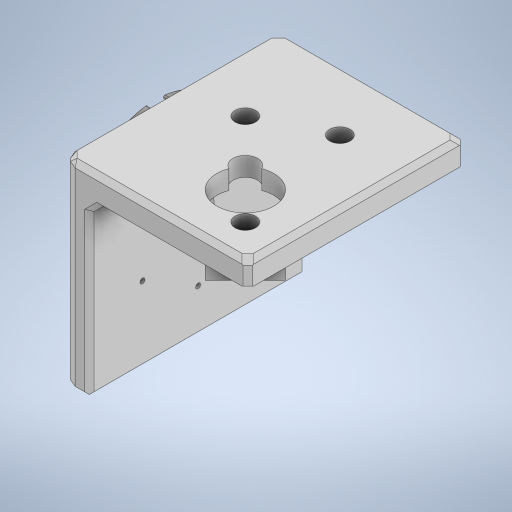
# Autodesk Inventor part: End_Effecto_Base
Saved by Autodesk Inventor 2023 (Build 270158000, 158)
## iProperties
Created: 2025-02-17
Part Number: End_Effecto_Base
Material: Generic
Document SubType Name: Modeling
Designer: Swoby
Density: 1 g/cm^3
Appearance: Default
Author: Swoby
Autodesk Inventor part; units mm, degrees
ref_plane "YZ Plane" through (0, 0, 0) normal (1, 0, 0) x (0, 1, 0)
ref_plane "XZ Plane" through (0, 0, 0) normal (0, 1, 0) x (-1, 0, 0)
ref_plane "XY Plane" through (0, 0, 0) normal (0, 0, 1) x (1, 0, 0)
sketch "Sketch1" plane through (0, 0, 0) normal (0, 0, 1) x (1, 0, 0)
  line L0 (0, 0) -> (-46, 0)
  line L1 (-46, 0) -> (-46, -38)
  line L2 (-46, -38) -> (-40, -38)
  line L3 (-40, -38) -> (-40, -6)
  line L4 (-40, -6) -> (0, -6)
  line L5 (0, -6) -> (0, 0)
  line L6 (-46, -38) -> (0, -38)
  line L7 (0, -38) -> (0, -42)
  line L8 (0, -42) -> (-46, -42)
  line L9 (-46, -42) -> (-46, -38)
  dimension "d0" = 38
  dimension "d1" = 40
  dimension "d2" = 6
  dimension "d3" = 6
  dimension "d62" = 4
  dimension "d63" = 32
  constraints: 20 end point, 6 perpendicular, 2 horizontal, 2 parallel, 1 collinear
  measures "d0" distance of L0.end L1.end
  measures "d1" distance of L3.end L4.end
  measures "d2" distance between parallel lines of L4 L0
  measures "d3" distance between parallel lines of L1 L3
  measures "d62" distance of L6.end L7.end
  measures "d63" distance between parallel lines of L4 L6
extrude "Extrusion1" add sketch "Sketch1" along normal blind 46
sketch "Sketch2" plane through (-46, 0, 0) normal (0, 1, 0) x (1, 0, 0)
  line L0 (46, 0) -> (0, 0) projected
  line L1 (0, 0) -> (0, -46) projected
  line L2 (46, -46) -> (0, -46) projected
  line L3 (46, 0) -> (46, -46) projected
  line L4 (26, 0) -> (26, -46) construction
  line L5 (46, -23) -> (26, -23) construction
  point P0 (26, -13)
  point P1 (26, -33)
  dimension "d6" = 20
  dimension "d7" = 10
  dimension "d8" = 10
  constraints: 4 end point, 4 point on line, 2 midpoint, 1 perpendicular
  measures "d6" distance between parallel lines of L4 L3
  measures "d7" distance from line of L5 point (26, -13)
  measures "d8" distance from line of point (26, -33) L5
sketch "Sketch3" plane through (-40, -6, 0) normal (0, -1, 0) x (1, 0, 0)
  circle A0 centre (20, 33) radius 6
  circle A1 centre (15.5452, 28.5452) radius 2.6
  line L0 (24.2426, 37.2426) -> (13.7067, 26.7067) construction
  line L1 (28.4853, 33) -> (20, 41.4853)
  line L2 (20, 41.4853) -> (3.9487, 25.434)
  line L3 (3.9487, 25.434) -> (12.434, 16.9487)
  line L4 (12.434, 16.9487) -> (28.4853, 33)
  line L5 (20, 33) -> (26, 33) construction
  line L6 (0, 0) -> (40, 0) projected
  line L7 (40, 0) -> (40, 46) projected
  line L8 (0, 46) -> (40, 46) projected
  line L9 (0, 0) -> (0, 46) projected
  point P0 (17.8741, 27.3892)
  point P1 (14.3892, 30.8741)
  point P2 (20, 13)
  dimension "d10" = 5.2
  dimension "d9" = 12
  dimension "d11" = 14.9
  dimension "d12" = 22.7
  dimension "d13" = 12
  dimension "d26" = 135
  constraints: 12 end point, 3 parallel, 2 point on circle, 2 point on line, 2 tangent, 1 centre point, 1 coincident, 1 horizontal, 1 perpendicular, 3 other
  measures "d9" diameter of A0
  measures "d11" distance of L0.start L0.end
  measures "d12" distance of L1.end L2.end
  measures "d13" distance of L2.end L3.end
  measures "d26" angle of L0 L5
extrude "Extrusion2" cut sketch "Sketch3" against normal through all contours A0 A1 | A1 A0 | A0 A1
extrude "Extrusion3" cut sketch "Sketch3" against normal blind 2 contours A0 A1 | A0 L1 L4 | A0 L2 L1 | L4 L3 L2 A0 A1 | A1 A0 | A0 A1
sketch "Sketch4" plane through (-40, -6, 0) normal (0, -1, 0) x (1, 0, 0)
  line L0 (3.9487, 25.434) -> (20, 41.4853) projected
  line L1 (20, 41.4853) -> (28.4853, 33) projected
  line L2 (28.4853, 33) -> (12.434, 16.9487) projected
  line L3 (12.434, 16.9487) -> (3.9487, 25.434) projected
  line L4 (0, 0) -> (40, 0) projected
  line L5 (40, 0) -> (40, 46) projected
  line L6 (0, 46) -> (40, 46) projected
  line L7 (0, 0) -> (0, 46) projected
  line L8 (28.4853, 33) -> (20, 41.4853)
  line L9 (3.9487, 25.434) -> (12.434, 16.9487)
  line L10 (12.434, 16.9487) -> (9.1106, 13.6253)
  line L11 (9.1106, 13.6253) -> (0.6253, 22.1106)
  line L12 (0.6253, 22.1106) -> (3.9487, 25.434)
  line L13 (28.4853, 33) -> (31.8087, 36.3234)
  line L14 (31.8087, 36.3234) -> (23.3234, 44.8087)
  line L15 (23.3234, 44.8087) -> (20, 41.4853)
  line L16 (31.8087, 36.3234) -> (20, 41.4853) construction
  line L17 (23.3234, 44.8087) -> (28.4853, 33) construction
  line L18 (12.434, 16.9487) -> (0.6253, 22.1106) construction
  line L19 (3.9487, 25.434) -> (9.1106, 13.6253) construction
  circle A0 centre (25.9043, 38.9043) radius 2.15
  circle A1 centre (6.5296, 19.5296) radius 2.15
  circle A2 centre (20, 13) radius 2.15
  circle A3 centre (20, 13) radius 4
  line L20 (23.3234, 44.8087) -> (24.0305, 45.5158)
  line L21 (24.0305, 45.5158) -> (32.5158, 37.0305)
  line L22 (32.5158, 37.0305) -> (31.8087, 36.3234)
  line L23 (0.6253, 22.1106) -> (0, 21.4853)
  line L24 (0, 21.4853) -> (0, 21.3216)
  line L25 (0, 21.3216) -> (8.4034, 12.9182)
  line L26 (8.4034, 12.9182) -> (9.1106, 13.6253)
  dimension "d28" = 4.7
  dimension "d29" = 4.7
  dimension "d30" = 12
  dimension "d31" = 4.3
  dimension "d32" = 4.3
  dimension "d35" = 4.3
  dimension "d36" = 8
  dimension "d76" = 1
  dimension "d77" = 1
  constraints: 38 end point, 6 collinear, 6 perpendicular, 4 centre point, 3 point on line, 2 coincident, 2 midpoint, 1 parallel
  measures "d28" distance of L2.end L10.end
  measures "d29" distance of L1.end L13.end
  measures "d30" distance of L13.end L14.end
  measures "d31" diameter of A0
  measures "d32" diameter of A1
  measures "d35" diameter of A2
  measures "d36" diameter of A3
  measures "d76" distance between parallel lines of L21 L14
  measures "d77" distance of L25.end L10.end
extrude "Extrusion4" add sketch "Sketch4" along normal blind 2.3 contours L3 L10 L11 L12 | L15 L14 L13 L1 | L11 L26 L25 L7 L23 | L20 L21 L22 L14 | A3
sketch "Sketch5" plane through (-20, -6, 41.35) normal (0, -1, 0) x (1, 0, 0)
  circle A0 centre (5.9043, -2.4457) radius 2.15 projected
  circle A1 centre (-13.4704, -21.8204) radius 2.15 projected
  circle A2 centre (0, -28.35) radius 2.15 projected
extrude "Extrusion5" cut sketch "Sketch5" against normal through all
sketch "Sketch6" plane through (-46, -38, 0) normal (-1, 0, 0) x (0, 0, 1)
  line L0 (0, 38) -> (0, 0) projected
  line L1 (0, 0) -> (46, 0) projected
  line L2 (46, 38) -> (46, 0) projected
  line L3 (0, 38) -> (46, 38) projected
  line L4 (0, 38) -> (46, 0) construction
  line L5 (0, 0) -> (46, 38) construction
  arc A0 (20.5564, 4.8718) -> (23, 2.9) centre (23, 5.4) ccw
  arc A1 (9.057, 10.95) -> (11.9864, 9.8197) centre (11.2221, 12.2) ccw
  line L6 (23, 2.9) -> (23, 19) construction
  line L7 (23, 19) -> (9.057, 10.95) construction
  circle A2 centre (23, 19) radius 8 construction
  line L8 (23, 19) -> (19, 12.0718) construction
  line L9 (19.0466, 11.8562) -> (20.5564, 4.8718)
  line L10 (18.79, 12.0044) -> (11.9864, 9.8197)
  arc A3 (19.0466, 11.8562) -> (18.79, 12.0044) centre (18.8511, 11.8139) ccw
  circle A4 centre (23, 5.4) radius 0.5
  circle A5 centre (34.7779, 12.2) radius 0.5
  arc A6 (34.0136, 9.8197) -> (36.943, 10.95) centre (34.7779, 12.2) ccw
  line L11 (27.21, 12.0044) -> (34.0136, 9.8197)
  arc A7 (27.21, 12.0044) -> (26.9534, 11.8562) centre (27.1489, 11.8139) ccw
  line L12 (26.9534, 11.8562) -> (25.4436, 4.8718)
  arc A8 (23, 2.9) -> (25.4436, 4.8718) centre (23, 5.4) ccw
  circle A9 centre (34.7779, 25.8) radius 0.5
  arc A10 (36.4572, 23.9479) -> (36.943, 27.05) centre (34.7779, 25.8) ccw
  line L13 (31.1634, 19.1482) -> (36.4572, 23.9479)
  arc A11 (31.1634, 19.1482) -> (31.1634, 18.8518) centre (31.2978, 19) ccw
  line L14 (31.1634, 18.8518) -> (36.4572, 14.0521)
  arc A12 (36.943, 10.95) -> (36.4572, 14.0521) centre (34.7779, 12.2) ccw
  circle A13 centre (23, 32.6) radius 0.5
  arc A14 (25.4436, 33.1282) -> (23, 35.1) centre (23, 32.6) ccw
  line L15 (26.9534, 26.1438) -> (25.4436, 33.1282)
  arc A15 (26.9534, 26.1438) -> (27.21, 25.9956) centre (27.1489, 26.1861) ccw
  line L16 (27.21, 25.9956) -> (34.0136, 28.1803)
  arc A16 (36.943, 27.05) -> (34.0136, 28.1803) centre (34.7779, 25.8) ccw
  circle A17 centre (11.2221, 25.8) radius 0.5
  arc A18 (11.9864, 28.1803) -> (9.057, 27.05) centre (11.2221, 25.8) ccw
  line L17 (18.79, 25.9956) -> (11.9864, 28.1803)
  arc A19 (18.79, 25.9956) -> (19.0466, 26.1438) centre (18.8511, 26.1861) ccw
  line L18 (19.0466, 26.1438) -> (20.5564, 33.1282)
  arc A20 (23, 35.1) -> (20.5564, 33.1282) centre (23, 32.6) ccw
  circle A21 centre (11.2221, 12.2) radius 0.5
  arc A22 (9.5428, 14.0521) -> (9.057, 10.95) centre (11.2221, 12.2) ccw
  line L19 (14.8366, 18.8518) -> (9.5428, 14.0521)
  arc A23 (14.8366, 18.8518) -> (14.8366, 19.1482) centre (14.7022, 19) ccw
  line L20 (14.8366, 19.1482) -> (9.5428, 23.9479)
  arc A24 (9.057, 27.05) -> (9.5428, 23.9479) centre (11.2221, 25.8) ccw
  circle A25 centre (23, 19) radius 3.4
  circle A26 centre (23, 19) radius 16
  point P0 (27, 12.0718)
  point P1 (31, 19)
  point P2 (27, 25.9282)
  point P3 (19, 25.9282)
  point P4 (15, 19)
  point P5 (23, 2.9)
  point P6 (36.943, 10.95)
  point P7 (36.943, 27.05)
  point P8 (23, 35.1)
  point P9 (9.057, 27.05)
  point P10 (8.7797, 11.6664)
  point P11 (9.5387, 10.3517)
  point P12 (22.241, 3.018)
  point P13 (23.759, 3.018)
  point P14 (36.4613, 10.3517)
  point P15 (37.2203, 11.6664)
  point P16 (37.2203, 26.3336)
  point P17 (36.4613, 27.6483)
  point P18 (23.759, 34.982)
  point P19 (22.241, 34.982)
  point P20 (9.5387, 27.6483)
  point P21 (8.7797, 26.3336)
  dimension "d44" = 16
  dimension "d39" = 5
  dimension "d40" = 5
  dimension "d41" = 60
  dimension "d42" = 16.1
  dimension "d43" = 16.1
  dimension "d45" = 30
  dimension "d46" = 0.2
  dimension "d47" = 1
  dimension "d48" = 360
  dimension "d53" = 6.8
  dimension "d81" = 32
  constraints: 36 point on circle, 34 end point, 26 centre point, 14 point on line, 10 coincident, 4 tangent, 1 midpoint, 1 vertical, 106 other
  measures "d39" diameter of A0
  measures "d40" diameter of A1
  measures "d41" angle of L7 L6
  measures "d42" distance of L6.start L7.start
  measures "d43" distance of L7.start L7.end
  measures "d45" angle of L6 L8
  measures "d46" radius of A3
  measures "d47" diameter of A4
  measures "d53" diameter of A25
  measures "d81" diameter of A26
extrude "Extrusion7" cut sketch "Sketch6" against normal blind 6 contours A4 | A5 | A9 | A13 | A17 | A21
extrude "Extrusion8" cut sketch "Sketch6" against normal through all contours A25
sketch "Sketch7" plane through (-40, -38, 0) normal (0, 1, 0) x (1, 0, 0)
  circle A0 centre (25.9043, -38.9043) radius 2.15 projected
  circle A1 centre (25.9043, -38.9043) radius 2.15 projected
  circle A2 centre (6.5296, -19.5296) radius 2.15 projected
  circle A3 centre (6.5296, -19.5296) radius 2.15 projected
  circle A4 centre (6.5296, -19.5296) radius 3.4
  circle A5 centre (25.9043, -38.9043) radius 3.4
  circle A6 centre (20, -13) radius 2.15 projected
  arc A7 (14.3892, -30.8741) -> (17.8741, -27.3892) centre (20, -33) ccw projected
  circle A8 centre (20, -13) radius 2.15
  circle A9 centre (20, -33) radius 2.15
  point P0 (40, 0)
  dimension "d64" = 6.8
  dimension "d65" = 6.8
  dimension "d74" = 4.3
  dimension "d75" = 4.3
  constraints: 4 centre point, 4 coincident
  measures "d64" diameter of A4
  measures "d65" diameter of A5
  measures "d74" diameter of A8
  measures "d75" diameter of A9
extrude "Extrusion9" cut sketch "Sketch7" against normal through all contours A0 | A2 | A4 | A5 A7 | A7 A5 | A6 | A9
chamfer "Chamfer3" distance 2 angle 45 9 edges at (0, -3, 46) (0, -40, 46) (-46, -21, 46) (-46, -21, 0) (0, -40, 0) (0, -3, 0) (-40, -38, 23) (-40, -6, 33.7426) (-40, -6, 10.6608)
chamfer "Chamfer4" distance 1 angle 45 36 edges at (-23, -42, 46) (-20, -38, 46) (-1, -42, 45) (-1, -38, 45) (0, -42, 23) (0, -38, 23) (-20, -38, 0) (-1, -38, 1) (-23, -42, 0) (-1, -42, 1) (-39, -37, 0) (-40, -22, 0) (-44, -21, 0) (-46, -42, 23) (-40, -22, 46) (-39, -37, 46) (-46, 0, 23) (-45, 0, 1) (-45, 0, 45) (-23, 0, 46) (-20, -6, 0) (-23, 0, 0) (-39, -7, 0) (-1, 0, 1) (0, 0, 23) (-1, 0, 45) (-1, -6, 1) (0, -6, 23) (-20, -6, 46) (-1, -6, 45) (-39, -7, 46) (-44, -21, 46) (-46, -21, 44) (-46, -21, 2) (-45, -42, 1) (-45, -42, 45)
chamfer "Chamfer5" distance 2 angle 45 1 edges at (-24, -6, 13)
extrude "Extrusion10" add sketch "Sketch6" along normal blind 3 contours L9 A3 L10 A1 A26 A22 L19 A23 L20 A24 A18 L17 A19 L18 A20 A14 L15 A15 L16 A16 A10 L13 A11 L14 A12 A6 L11 A7 L12 A8 A0 | A0 A26 A1 L10 A3 L9 | A8 L12 A7 L11 A6 A26 | A26 A24 L20 A23 L19 A22 | A12 L14 A11 L13 A10 A26 | A26 A20 L18 A19 L17 A18 | A26 A16 L16 A15 L15 A14
extrude "Extrusion11" cut sketch "Sketch6" along normal blind 3 and the other way blind 1 contours L9 A3 L10 A1 A26 A22 L19 A23 L20 A24 A18 L17 A19 L18 A20 A14 L15 A15 L16 A16 A10 L13 A11 L14 A12 A6 L11 A7 L12 A8 A0
fillet "Fillet1" radius 0.3 12 edges at (-47.5, -3.018, 22.241) (-47.5, -3.018, 23.759) (-47.5, -10.3517, 9.5387) (-47.5, -11.6664, 8.7797) (-47.5, -26.3336, 8.7797) (-47.5, -27.6483, 9.5387) (-47.5, -34.982, 22.241) (-47.5, -34.982, 23.759) (-47.5, -26.3336, 37.2203) (-47.5, -27.6483, 36.4613) (-47.5, -10.3517, 36.4613) (-47.5, -11.6664, 37.2203)
sketch "Sketch8" plane through (0, 0, 46) normal (0, 0, 1) x (1, 0, 0)
  line L0 (-2, -5) -> (-38.4142, -5) projected
  line L1 (-2, -1) -> (-2, -5) projected
  line L2 (-43, -1) -> (-2, -1) projected
  line L3 (-43, -41) -> (-43, -1) projected
  line L4 (-2, -41) -> (-43, -41) projected
  line L5 (-2, -39) -> (-2, -41) projected
  line L6 (-38.4142, -39) -> (-2, -39) projected
  line L7 (-41, -36.4142) -> (-38.4142, -39) projected
  line L8 (-41, -7.5858) -> (-41, -36.4142) projected
  line L9 (-38.4142, -5) -> (-41, -7.5858) projected
  line L10 (-7.4842, -6) -> (-7.4842, -8.3) projected
  line L11 (0, -5) -> (0, -1) projected
  line L12 (-2.4142, 0) -> (-43.5858, 0) projected
  line L13 (-43.5858, -42) -> (-2.4142, -42) projected
  line L14 (-1, 0) -> (-2.4142, 0) projected
  line L15 (-1, 0) -> (-2.4142, 0) projected
  line L16 (-2, -1) -> (-2.4142, 0) projected
  line L17 (-2, -1) -> (0, -1) projected
  line L18 (0, -1) -> (-1, 0) projected
  line L19 (-1, -6) -> (0, -5) projected
  line L20 (-2.4142, -6) -> (-1, -6) projected
  line L21 (-15.4537, -6) -> (-15.9695, -5.4842) projected
  line L22 (-15.4537, -6) -> (-2.4142, -6) projected
  line L23 (-2.4142, -6) -> (-2, -5) projected
  line L24 (-2, -5) -> (-38.4142, -5) projected
  line L25 (-38.4142, -5) -> (-38, -6) projected
  line L26 (-38, -6) -> (-16.4853, -6) projected
  line L27 (-15.9695, -5.4842) -> (-16.4853, -6) projected
  line L28 (0, -5) -> (-2, -5) projected
  line L29 (0, -5) -> (0, -1) projected
  line L30 (-2, -1) -> (0, -1) projected
  line L31 (-2, -1) -> (-2, -5) projected
  line L32 (-7.4842, -6) -> (-7.4842, 0) construction
  line L33 (-7.4842, 0) -> (-6.4842, -1)
  line L34 (-6.4842, -1) -> (-6.4842, -5)
  line L35 (-7.4842, -6) -> (-6.4842, -5)
  line L36 (-38.4142, -39) -> (-2, -39) projected
  line L37 (-2, -39) -> (-2.4142, -38) projected
  line L38 (-2.4142, -38) -> (-38, -38) projected
  line L39 (-38.4142, -39) -> (-38, -38) projected
  line L40 (-1, -38) -> (-2.4142, -38) projected
  line L41 (-2, -39) -> (-2.4142, -38) projected
  line L42 (-2, -39) -> (0, -39) projected
  line L43 (0, -39) -> (-1, -38) projected
  line L44 (-2, -39) -> (0, -39) projected
  line L45 (-2, -39) -> (-2, -41) projected
  line L46 (0, -41) -> (-2, -41) projected
  line L47 (0, -41) -> (0, -39) projected
  line L48 (0, -41) -> (-2, -41) projected
  line L49 (-2.4142, -42) -> (-2, -41) projected
  line L50 (-2.4142, -42) -> (-1, -42) projected
  line L51 (-1, -42) -> (0, -41) projected
  line L52 (-7.4842, -38) -> (-6.4842, -39)
  line L53 (-6.4842, -39) -> (-6.4842, -41)
  line L54 (-7.4842, -42) -> (-6.4842, -41)
  line L55 (-40, -36) -> (-40, -8) projected
  line L56 (-40, -36) -> (-40, -41)
  line L57 (-40, -41) -> (-41, -42)
  line L58 (-41, -36.4142) -> (-38.4142, -39) projected
  line L59 (-38.4142, -39) -> (-38, -38) projected
  line L60 (-38, -38) -> (-40, -36) projected
  line L61 (-41, -36.4142) -> (-40, -36) projected
  point P0 (0, 0)
  point P1 (0, -39)
  point P2 (-2.4142, -42)
  point P3 (-2.4142, -6)
  point P4 (-40, -37.4142)
  dimension "d89" = 1
  dimension "d90" = 1
  dimension "d91" = 1
  dimension "d92" = 1
  dimension "d98" = 45
  constraints: 18 end point, 13 point on line, 2 perpendicular, 2 vertical
  measures "d89" distance between parallel lines of L12 L2
  measures "d90" distance between parallel lines of L34 L32
  measures "d91" distance from line of L52.start L53
  measures "d92" distance from line of L47 L40.start
  measures "d98" angle of L4 L57
extrude "Extrusion12" cut sketch "Sketch8" against normal through all contours L23 L22 L35 L0 | L0 L34 L2 L1 | L28 L19 L20 L23 | L1 L17 L11 L28 | L2 L33 L12 L16 | L16 L14 L18 L17 | L56 L60 L39 L7 | L7 L6 L53 L4 L56 | L4 L54 L13 L57 | L39 L38 L52 L6 | L53 L6 L5 L4 | L4 L49 L13 L54 | L52 L38 L37 L6 | L5 L42 L47 L46 | L46 L51 L50 L49 | L37 L40 L43 L42
chamfer "Chamfer6" distance 1 angle 45 8 edges at (-6.4842, -3, 46) (-6.9842, -0.5, 45.5) (-6.9842, -5.5, 45.5) (-6.4842, -3, 0) (-6.9842, -0.5, 0.5) (-6.9842, -5.5, 0.5) (-40, -39.2071, 46) (-40, -39.2071, 0)
equation "\"d8\" = d7"
equation "\"d43\" = d42"
equation "\"d45\" = 0.5 * d41"
body "Solid1"
